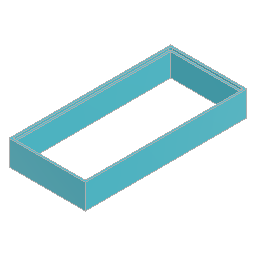
Pencil-Holder (Autodesk Fusion 360 design; units mm, degrees)
Autodesk Fusion 360 part; units mm, degrees
sketch "sketch 358" plane through (0, 0, 3.175) normal (0, 0, 1) x (-1, 0, 0)
  arc A0 (-283.15, 173.942) -> (-281.1, 175.992) centre (-281.1, 173.942) cw
  line L0 (-281.1, 175.992) -> (-205.1, 175.992)
  arc A1 (-205.1, 175.992) -> (-203.05, 173.942) centre (-205.1, 173.942) cw
  line L1 (-203.05, 173.942) -> (-203.05, 3.992)
  arc A2 (-203.05, 3.992) -> (-205.1, 1.942) centre (-205.1, 3.992) cw
  line L2 (-205.1, 1.942) -> (-281.1, 1.942)
  arc A3 (-281.1, 1.942) -> (-283.15, 3.992) centre (-281.1, 3.992) cw
  line L3 (-283.15, 3.992) -> (-283.15, 173.942)
  line L4 (-201.1, 0) -> (-285.1, 0)
  line L5 (-201.1, 0) -> (-285.1, 0)
  line L6 (-201.1, 177.942) -> (-201.1, 0)
  line L7 (-285.1, 177.942) -> (-201.1, 177.942)
  line L8 (-285.1, 177.942) -> (-201.1, 177.942)
  line L9 (-285.1, 0) -> (-285.1, 177.942)
extrude "Extrude1" add sketch "sketch 358" along normal blind 27.5
sketch "sketch 414" plane through (0, 0, 3.175) normal (0, 0, 1) x (-1, 0, 0)
  line L0 (-281.1, 173.942) -> (-205.1, 173.942)
  line L1 (-205.1, 173.942) -> (-205.1, 4)
  line L2 (-205.1, 4) -> (-281.1, 4)
  line L3 (-281.1, 4) -> (-281.1, 173.942)
  arc A0 (-281.1, 175.992) -> (-283.15, 173.942) centre (-281.1, 173.942) ccw
  line L4 (-283.15, 173.942) -> (-283.15, 3.992)
  arc A1 (-283.15, 3.992) -> (-281.1, 1.942) centre (-281.1, 3.992) ccw
  line L5 (-281.1, 1.942) -> (-205.1, 1.942)
  arc A2 (-205.1, 1.942) -> (-203.05, 3.992) centre (-205.1, 3.992) ccw
  line L6 (-203.05, 3.992) -> (-203.05, 173.942)
  arc A3 (-203.05, 173.942) -> (-205.1, 175.992) centre (-205.1, 173.942) ccw
  line L7 (-205.1, 175.992) -> (-281.1, 175.992)
extrude "Extrude2" add sketch "sketch 414" along normal blind 25
